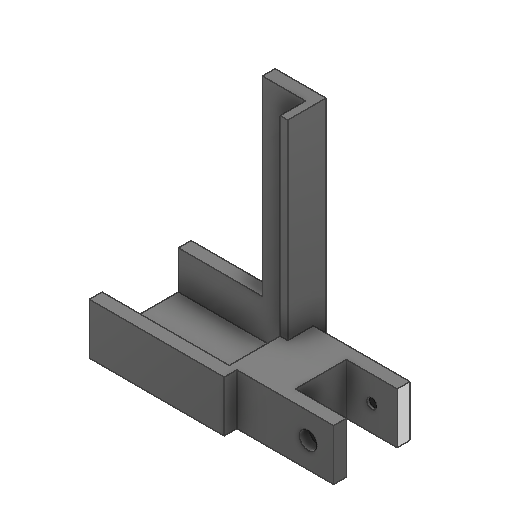
# Autodesk Inventor part: PowerSupplyAttachTop
Saved by Autodesk Inventor 2025.2 (Build 292293000, 293)
## iProperties
Created: 2026-03-03
Part Number: PowerSupplyAttachTop
Material: Generic
Document SubType Name: Modeling
Designer: rolan
Density: 1 g/cm^3
Appearance: Default
Author: rolan
Autodesk Inventor part; units mm, degrees
ref_plane "YZ Plane" through (0, 0, 0) normal (1, 0, 0) x (0, 1, 0)
ref_plane "XZ Plane" through (0, 0, 0) normal (0, 1, 0) x (-1, 0, 0)
ref_plane "XY Plane" through (0, 0, 0) normal (0, 0, 1) x (1, 0, 0)
sketch "Sketch1" plane through (0, 0, 0) normal (0, 1, 0) x (-1, 0, 0)
  line L0 (0, 0) -> (50, 0)
  line L1 (50, 0) -> (50, -40)
  line L2 (50, -40) -> (0, -40)
  line L3 (0, -40) -> (0, 0)
  line L4 (0, -5) -> (-41, -5)
  line L5 (-41, -5) -> (-41, -10)
  line L6 (-41, -10) -> (0, -10)
  line L7 (0, -10) -> (0, -5)
  line L8 (0, -30) -> (-41, -30)
  line L9 (-41, -30) -> (-41, -35)
  line L10 (-41, -35) -> (0, -35)
  line L11 (0, -35) -> (0, -30)
  line L12 (0, 0) -> (-3, 0)
  line L13 (-3, 0) -> (-3, -5)
  line L14 (-3, -5) -> (0, -5)
  line L15 (0, -5) -> (0, 0)
  line L16 (0, -40) -> (-3, -40)
  line L17 (-3, -40) -> (-3, -35)
  line L18 (-3, -35) -> (0, -35)
  line L19 (0, -35) -> (0, -40)
  line L20 (0, -10) -> (-21, -10)
  line L21 (-21, -10) -> (-21, -30)
  line L22 (-21, -30) -> (0, -30)
  line L23 (0, -30) -> (0, -10)
  point P0 (0, -10)
  point P1 (-21, -10)
  dimension "d0" = 50
  dimension "d1" = 40
  dimension "d2" = 41
  dimension "d3" = 41
  dimension "d4" = 5
  dimension "d5" = 5
  dimension "d6" = 5
  dimension "d7" = 5
  dimension "d8" = 3
  dimension "d9" = 5
  dimension "d39" = 21
  constraints: 48 end point, 12 parallel, 6 horizontal, 6 perpendicular, 4 point on line
  measures "d0" distance of L1.end L2.end
  measures "d1" distance of L0.end L1.end
  measures "d2" distance of L4.start L4.end
  measures "d3" distance of L8.start L8.end
  measures "d4" distance of L4.end L5.end
  measures "d5" distance of L8.end L9.end
  measures "d6" distance from line of L2.end L10
  measures "d7" distance from line of L0.start L4
  measures "d8" distance of L14.end L13.end
  measures "d9" distance of L13.end L12.end
  measures "d39" distance between parallel lines of L23 L21
extrude "Extrusion1" add sketch "Sketch1" along normal blind 20
sketch "Sketch2" plane through (0, 20, 0) normal (0, 1, 0) x (1, 0, 0)
  line L0 (-50, 40) -> (-50, 0) projected
  line L1 (-50, 5) -> (0, 5)
  line L2 (0, 5) -> (0, 35)
  line L3 (0, 35) -> (-50, 35)
  line L4 (-50, 35) -> (-50, 5)
  line L5 (3, 40) -> (-50, 40) projected
  point P0 (0, 0)
  point P1 (-50, 35)
  dimension "d12" = 50
  dimension "d13" = 30
  dimension "d26" = 5
  constraints: 8 end point, 2 parallel, 1 horizontal, 1 perpendicular, 1 point on line
  measures "d12" distance of L3.end L2.end
  measures "d13" distance of L2.end L1.end
  measures "d26" distance between parallel lines of L5 L3
extrude "Extrusion2" cut sketch "Sketch2" against normal blind 15
sketch "Sketch3" plane through (3, 0, -5) normal (0, 0, 1) x (1, 0, 0)
  circle A0 centre (28, 10) radius 3.5
  line L0 (38, 0) -> (38, 20) projected
  line L1 (0, 20) -> (38, 20) projected
  point P0 (-3, 0)
  point P1 (19, 20)
  dimension "d16" = 10
  dimension "d17" = 10
  dimension "d20" = 7
  constraints: 1 centre point, 1 midpoint
  measures "d16" distance from line of L0 A0.centre
  measures "d17" vertical distance of point (19, 20) A0.centre
  measures "d20" diameter of A0
extrude "Extrusion3" cut sketch "Sketch3" against normal blind 4
sketch "Sketch4" plane through (41, 0, -35) normal (0, 0, -1) x (-1, 0, 0)
  circle A0 centre (10, 10) radius 3.5 projected
  circle A1 centre (10, 10) radius 3.5 projected
  point P0 (41, 0)
extrude "Extrusion4" cut sketch "Sketch4" against normal blind 4
sketch "Sketch5" plane through (31, 10, -31) normal (0, 0, -1) x (-1, 0, 0)
  circle A0 centre (0, 0) radius 2
  point P0 (31, -10)
  dimension "d23" = 4
  constraints: 1 centre point
  measures "d23" diameter of A0
extrude "Extrusion5" cut sketch "Sketch5" against normal through all
sketch "Sketch6" plane through (0, 0, 0) normal (0, -1, 0) x (1, 0, 0)
  circle A0 centre (-25, -17.5) radius 3.5
  line L0 (0, -5) -> (-50, -5) projected
  point P0 (0, 0)
  point P1 (-50, -35)
  point P2 (0, -35)
  dimension "d27" = 7
  dimension "d29" = 25
  dimension "d44" = 12.5
  constraints: 1 centre point
  measures "d27" diameter of A0
  measures "d29" horizontal distance of A0.centre point (0, -35)
  measures "d44" distance from line of L0 A0.centre
extrude "Extrusion6" cut sketch "Sketch6" against normal blind 4
sketch "Sketch7" plane through (-25, 4, -17.5) normal (0, -1, 0) x (1, 0, 0)
  circle A0 centre (0, 0) radius 2
  point P0 (25, 17.5)
  dimension "d32" = 4
  constraints: 1 centre point
  measures "d32" diameter of A0
extrude "Extrusion7" cut sketch "Sketch7" against normal blind 4
sketch "Sketch9" plane through (0, 20, 0) normal (0, 1, 0) x (1, 0, 0)
  line L0 (3, 35) -> (3, 40) projected
  line L1 (-50, 35) -> (0, 35) projected
  line L2 (3, 40) -> (-17, 40)
  line L3 (-17, 40) -> (-17, 35)
  line L4 (-17, 35) -> (3, 35)
  line L5 (3, 35) -> (3, 40)
  line L6 (0, 35) -> (0, 5) projected
  line L7 (3, 35) -> (0, 35)
  line L8 (0, 35) -> (0, 25)
  line L9 (0, 25) -> (3, 25)
  line L10 (3, 25) -> (3, 35)
  point P0 (0, 0)
  point P1 (0, 15)
  dimension "d40" = 20
  dimension "d41" = 10
  constraints: 16 end point, 4 parallel, 2 horizontal, 2 perpendicular, 2 point on line
  measures "d40" distance of L4.end L3.end
  measures "d41" distance of L8.end L7.end
extrude "Extrusion9" add sketch "Sketch9" along normal blind 75
body "Solid1"
